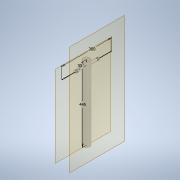
# Autodesk Inventor part: FrontWheelHandle
Saved by Autodesk Inventor 2022.2 (Build 262287000, 287)
## iProperties
Created: 2022-04-15
Part Number: FrontWheelHandle
Material: Aluminum 6061
Document SubType Name: Modeling
Designer: foriw
Density: 2.7 g/cm^3
Appearance: Aluminum - Flat
Author: foriw
Autodesk Inventor part; units mm, degrees
ref_plane "XZ Plane" through (0, 0, 0) normal (0, 1, 0) x (-1, 0, 0)
ref_plane "XY Plane" through (0, 0, 0) normal (0, 0, 1) x (1, 0, 0)
sketch "Sketch1" plane through (0, 0, 0) normal (1, 0, 0) x (0, 1, 0)
  line L0 (0, 0) -> (445, 0)
  line L1 (415, -150) -> (415, 150)
  point P0 (415, 0)
  dimension "d0" = 445
  dimension "d1" = 30
  dimension "d2" = 300
  constraints: 4 end point, 1 horizontal, 1 midpoint, 1 point on line, 1 vertical
  measures "d0" distance of L0.start L0.end
  measures "d1" distance of L0.end point (415, 0)
  measures "d2" distance of L1.start L1.end
sketch "Sketch2" plane through (0, 0, 0) normal (0, 1, 0) x (-1, 0, 0)
  circle A0 centre (0, 0) radius 21
  circle A1 centre (0, 0) radius 17.65
  dimension "d3" = 42
  dimension "d18" = 35.3
  constraints: 2 centre point, 1 coincident
  measures "d3" diameter of A0
  measures "d18" diameter of A1
ref_plane "Work Plane1" through (0, 415, 0) normal (0, 0, 1) x (1, 0, 0)
sketch "Sketch3" plane through (0, 415, 0) normal (0, 0, 1) x (1, 0, 0)
  circle A0 centre (0, 0) radius 9
  circle A1 centre (0, 0) radius 5.5
  point P0 (0, -415)
  dimension "d5" = 18
  dimension "d6" = 3.5
  constraints: 2 centre point
  measures "d5" diameter of A0
  measures "d6" radial gap between concentric circles of A0 A1
extrude "Extrusion1" add sketch "Sketch3" along normal mid plane 140
extrude "Extrusion2" add sketch "Sketch2" along normal up to surface (445 mm away)
ref_plane "Work Plane2" through (64, 0, 0) normal (1, 0, 0) x (0, 1, 0)
sketch "Sketch4" plane through (64, 0, 0) normal (1, 0, 0) x (0, 1, 0)
  circle A0 centre (16, 0) radius 2
  circle A1 centre (45, 0) radius 2
  line L0 (43, 7.4424) -> (43, -6.8322)
  line L1 (18, 4.2123) -> (18, -2.7864)
  line L2 (14, 2.9252) -> (14, -3.9898)
  line L3 (0, -21) -> (0, 21) projected
  point P0 (0, 0)
  dimension "d12" = 4
  dimension "d13" = 4
  dimension "d14" = 25
  dimension "d15" = 14
  constraints: 6 end point, 3 tangent, 3 vertical, 2 centre point
  measures "d12" diameter of A0
  measures "d13" diameter of A1
  measures "d14" distance between parallel lines of L0 L1
  measures "d15" distance between parallel lines of L3 L2
extrude "Extrusion3" cut sketch "Sketch4" against normal blind 54.75
ref_plane "Work Plane3" through (-21, 0, 0) normal (1, 0, 0) x (0, 1, 0)
sketch "Sketch5" plane through (-21, 0, 0) normal (1, 0, 0) x (0, 1, 0)
  line L0 (313.5, -6.5) -> (387, -6.5)
  arc A0 (387, -6.5) -> (387, 6.5) centre (387, 0) ccw
  line L1 (387, 6.5) -> (313.5, 6.5)
  arc A1 (313.5, 6.5) -> (313.5, -6.5) centre (313.5, 0) ccw
  line L2 (393.5, 48.7813) -> (393.5, 74.201)
  line L3 (307, 48.7813) -> (307, 80.9156)
  line L4 (445, 21) -> (445, -21) projected
  line L5 (441.5, -1.7269) -> (441.5, 5.9904)
  line L6 (445, -17.65) -> (445, 17.65) projected
  line L7 (445, -1.5) -> (446.3982, -1.5)
  line L8 (446.3982, -1.5) -> (443, -1.5)
  arc A2 (443, 1.5) -> (443, -1.5) centre (443, 0) ccw
  line L9 (443, 1.5) -> (445, 1.5)
  point P0 (0, 0)
  point P1 (350.25, 6.5)
  point P2 (350.25, -6.5)
  dimension "d19" = 86.5
  dimension "d20" = 13
  dimension "d21" = 3.5
  dimension "d22" = 3
  dimension "d23" = 48
  constraints: 16 end point, 9 tangent, 6 point on circle, 3 centre point, 3 horizontal, 3 point on line, 3 vertical, 2 midpoint, 1 perpendicular
  measures "d19" distance between parallel lines of L3 L2
  measures "d20" distance of point (350.25, 6.5) point (350.25, -6.5)
  measures "d21" distance between parallel lines of L6 L5
  measures "d22" distance from line of L9.start L7
  measures "d23" distance between parallel lines of L2 L5
extrude "Extrusion4" cut sketch "Sketch5" along normal blind 10
sketch "Sketch6" plane through (-21, 0, 0) normal (1, 0, 0) x (0, 1, 0)
  circle A0 centre (384.25, 0) radius 2.25
  circle A1 centre (322.25, 0) radius 2.25
  line L0 (386.5, -4.1522) -> (386.5, 4.2632)
  line L1 (445, 21) -> (445, -21) projected
  line L2 (324.5, -4.1522) -> (324.5, 4.2632)
  point P0 (0, 0)
  point P1 (445, -1.5)
  point P2 (445, 1.5)
  dimension "d26" = 4.5
  dimension "d27" = 4.5
  dimension "d28" = 58.5
  dimension "d29" = 120.5
  constraints: 4 end point, 2 centre point, 2 tangent, 2 vertical
  measures "d26" diameter of A0
  measures "d27" diameter of A1
  measures "d28" distance between parallel lines of L1 L0
  measures "d29" distance between parallel lines of L1 L2
extrude "Extrusion5" cut sketch "Sketch6" along normal through all
chamfer "Chamfer1" distance 2 angle 45 2 edges at (21, 382, 0) (21, 320, 0)
thread "Thread1" size "M18x2.5" class "6g" standard "ANSI Metric M Profile" length 14
thread "Thread2" size "M18x2.5" class "6g" standard "ANSI Metric M Profile" length 14
equation "\"d13\" = d12"
body "Solid1"
